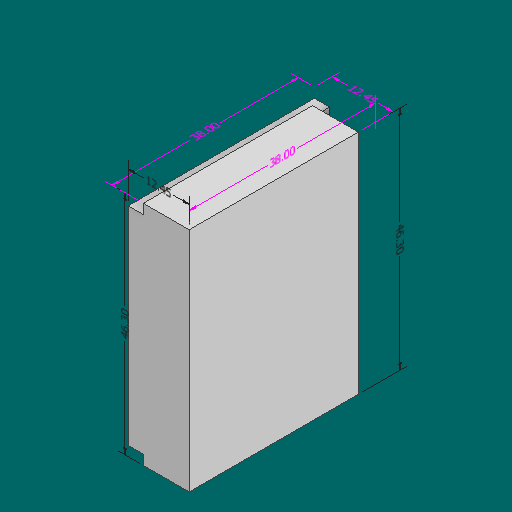
# Autodesk Inventor part: MiniBB_SD_PD
Saved by Autodesk Inventor 2025.2 (Build 292293000, 293)
## iProperties
Created: 2025-04-19
Part Number: MiniBB_SD_PD
Material: Generic
Document SubType Name: Modeling
Designer: Matt Caldwell
Density: 1 g/cm^3
Appearance: Default
Author: Matt Caldwell
Autodesk Inventor part; units mm, degrees
ref_plane "YZ Plane" through (0, 0, 0) normal (1, 0, 0) x (0, 1, 0)
ref_plane "XZ Plane" through (0, 0, 0) normal (0, 1, 0) x (-1, 0, 0)
ref_plane "XY Plane" through (0, 0, 0) normal (0, 0, 1) x (1, 0, 0)
sketch "Sketch1" plane through (0, 0, 0) normal (0, 1, 0) x (-1, 0, 0)
  line L0 (-10.0497, 12.7691) -> (-22.4997, 12.7691)
  line L1 (-22.4997, 12.7691) -> (-22.4997, -25.2309)
  line L2 (-22.4997, -25.2309) -> (-10.0497, -25.2309)
  line L3 (-10.0497, -25.2309) -> (-10.0497, 12.7691)
  dimension "d0" = 12.45
  dimension "d1" = 38
  constraints: 8 end point, 2 parallel, 1 horizontal, 1 perpendicular
  measures "d0" distance between parallel lines of L1 L3
  measures "d1" distance between parallel lines of L2 L0
extrude "Extrusion1" add sketch "Sketch1" along normal blind 46.3
sketch "Sketch2" plane through (0, 46.3, 0) normal (0, 1, 0) x (1, 0, 0)
  line L0 (13.1497, -12.7691) -> (13.1497, 21.7309)
  line L1 (13.1497, 21.7309) -> (22.4997, 21.7309)
  line L2 (22.4997, 21.7309) -> (22.4997, 25.2309)
  line L3 (22.4997, 25.2309) -> (10.0497, 25.2309) projected
  line L4 (10.0497, 25.2309) -> (10.0497, -12.7691) projected
  line L5 (10.0497, 25.2309) -> (10.0497, -12.7691)
  line L6 (10.0497, -12.7691) -> (13.1497, -12.7691)
  line L7 (13.1497, 21.7309) -> (22.4997, 21.7309)
  point P0 (0, 0)
  point P1 (22.4997, -12.7691)
  point P2 (17.8247, -12.7691)
  point P3 (17.8247, 21.7309)
  constraints: 12 end point, 2 collinear, 1 midpoint, 1 perpendicular
extrude "Extrusion2" cut sketch "Sketch2" against normal blind 2
sketch "Sketch3" plane through (0, 44.3, 0) normal (0, 1, 0) x (1, 0, 0)
  line L0 (22.4997, -12.7691) -> (22.4997, 25.2309) projected
  line L1 (13.1497, 21.7309) -> (13.1497, -12.7691) projected
  line L2 (22.4997, 21.7309) -> (13.1497, 21.7309)
  line L3 (13.1497, 21.7309) -> (13.1497, 25.2309)
  line L4 (22.4997, 25.2309) -> (10.0497, 25.2309) projected
  line L5 (22.4997, 25.2309) -> (22.4997, 21.7309)
  point P0 (0, 0)
  constraints: 6 end point, 2 perpendicular, 2 point on line, 1 parallel
extrude "Extrusion3" cut sketch "Sketch3" against normal blind 44.8625
sketch "Sketch5" plane through (0, 0, 0) normal (0, -1, 0) x (1, 0, 0)
  line L0 (10.0497, -25.2309) -> (10.0497, 12.7691) projected
  line L1 (13.1497, -25.2309) -> (10.0497, -25.2309) projected
  line L2 (10.0497, -25.2309) -> (13.1497, -25.2309)
  line L3 (13.1497, -21.7309) -> (13.1497, 12.7691) projected
  line L4 (13.1497, -25.2309) -> (13.1497, 12.7691)
  line L5 (13.1497, 12.7691) -> (10.0497, 12.7691)
  line L6 (10.0497, 12.7691) -> (10.0497, -25.2309)
  point P0 (0, 0)
  constraints: 8 end point, 2 perpendicular, 1 collinear, 1 horizontal
extrude "Extrusion4" cut sketch "Sketch5" against normal blind 2
body "Solid1"
